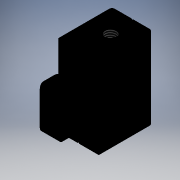
# Autodesk Inventor part: HCBRB8
Saved by Autodesk Inventor 2017.3 (Build 213256000, 256)
## iProperties
Part Number: HCBRB8
Material: Generic
Catalog Web Link: www.cadenas.de
Description: HCBR, HCBRB-Panel Support Brackets - Resin Type - for Center Mounting (One-Touch Mounting)
Vendor: MISUMI
Document SubType Name: Modeling
Designer: partserver
Manufacturer: MISUMI
Mass: 8.4889 g
Surface Area: 43.6631 cm^2
Volume: 8.4889 cm^3
Density: 1 g/cm^3
Appearance: PSOLRGB-0-0-0
Category: PARTsolutions
Company: MISUMI
Title: HCBRB8
Author: Cadenas PARTsolutions
Comments: Panel Support Brackets - Resin Type - for Center Mounting (One-Touch Mounting)
PSOL_IDENT_0: {$CADENAS_DATA\23d-libs\misumi\metric\39_accessories_for_al_extrusions\hcbr.prj},162 {VTYP=3D},{NB=H
PSOL_IDENT_1: CBRB8},{LINA=HCBRB8},{NN=HCBR, HCBRB},{DATE=08.06.2021 06:07:33},{GEOMDATE=12.08.2016 06:28:00},{VER
PSOL_IDENT_2: SION=},{LINEID=40},{WBVAR=COLOR},{WBNUMERIC=}  {NB=HCBRB8},{LINA=HCBRB8},{KT=DUMMY},{PN=HCBRB8},{COL
PSOL_IDENT_3: OR=B},{TS=HCBR},{MAT=Polyamide},{NO=8},{MASS=10.9},{A=30},{DIFF=5},{COL=0.00,0.00,0.00,0.00},{M=5},{
PSOL_IDENT_4: KDM=4.134}
NB: HCBRB8
NN: HCBR, HCBRB
NT: Panel Support Brackets - Resin Type - for Center Mounting (One-Touch Mounting)
NBSYN: $PN.
LINA: HCBRB8
CATALOG: Misumi
PN: HCBRB8
COLOR: Black
MAT: Polyamide
NO: 8
MASS: 10.9
A: 30
DIFF: 5
SUPPLIER: MISUMI
ARTICLENO: HCBRB8
BOMINFO: HCBRB8
CREATOR: CADENAS GmbH
Autodesk Inventor part; units mm, degrees
ref_plane "YZ Plane" through (0, 0, 0) normal (1, 0, 0) x (0, 1, 0)
ref_plane "XZ Plane" through (0, 0, 0) normal (0, 1, 0) x (-1, 0, 0)
ref_plane "XY Plane" through (0, 0, 0) normal (0, 0, 1) x (1, 0, 0)
sketch "Sketch_1" plane through (0, 0, 0) normal (0, 0, 1) x (1, 0, 0)
  line L0 (0, 28.85) -> (0, 9.95)
  line L1 (0, 9.95) -> (15, 9.95)
  line L2 (15, 9.95) -> (15, 28.85)
  arc A0 (15, 28.85) -> (14, 29.85) centre (14, 28.85) ccw
  line L3 (14, 29.85) -> (1, 29.85)
  arc A1 (1, 29.85) -> (0, 28.85) centre (1, 28.85) ccw
  constraints: 8 end point, 4 point on circle, 2 centre point
extrude "Extrusion1" add sketch "Sketch_1" against normal blind 30
sketch "Sketch_6" plane through (7.5, 0, 0) normal (1, 0, 0) x (0, 0, -1)
  line L0 (0, 21.4) -> (35, 21.4)
  line L1 (35, 21.4) -> (35, 18.15)
  line L2 (35, 18.15) -> (34.5, 18.65)
  line L3 (34.5, 18.65) -> (0.5, 18.65)
  line L4 (0.5, 18.65) -> (0, 18.15)
  line L5 (0, 18.15) -> (0, 21.4)
  line L6 (0, 21.4) -> (35, 21.4)
  constraints: 14 end point
revolve "Revolution1" cut sketch "Sketch_6" angle 360 about axis through (7.5, 21.4, 0) along (0, 0, 1)
sketch "Sketch_4" plane through (7.5, 0, 0) normal (1, 0, 0) x (0, 0, -1)
  line L0 (0, 22.5) -> (35, 22.5)
  line L1 (35, 22.5) -> (35, 19.25)
  line L2 (35, 19.25) -> (34.5, 19.75)
  line L3 (34.5, 19.75) -> (0.5, 19.75)
  line L4 (0.5, 19.75) -> (0, 19.25)
  line L5 (0, 19.25) -> (0, 22.5)
  line L6 (0, 22.5) -> (35, 22.5)
  constraints: 14 end point
revolve "Revolution2" cut sketch "Sketch_4" angle 360 about axis through (7.5, 22.5, 0) along (0, 0, 1)
sketch "Sketch_8" plane through (0, 21.95, 0) normal (0, 1, 0) x (1, 0, 0)
  line L0 (4.25, 0) -> (10.75, 0)
  line L1 (10.75, 0) -> (10.25, 0.5)
  line L2 (10.25, 0.5) -> (10.25, 34.5)
  line L3 (10.25, 34.5) -> (10.75, 35)
  line L4 (10.75, 35) -> (4.25, 35)
  line L5 (4.25, 35) -> (4.75, 34.5)
  line L6 (4.75, 34.5) -> (4.75, 0.5)
  line L7 (4.75, 0.5) -> (4.25, 0)
  constraints: 16 end point
extrude "Extrusion2" cut sketch "Sketch_8" along normal mid plane 1.1
sketch "Sketch_10" plane through (0, 0, -0.5) normal (0, 0, 1) x (1, 0, 0)
  arc A0 (4.75, 21.4) -> (10.25, 21.4) centre (7.5, 21.4) ccw
  line L0 (10.25, 21.4) -> (10.25, 22.5)
  arc A1 (10.25, 22.5) -> (4.75, 22.5) centre (7.5, 22.5) ccw
  line L1 (4.75, 22.5) -> (4.75, 21.4)
  constraints: 4 end point, 4 point on circle, 2 centre point
extrude "Extrusion3" add sketch "Sketch_10" against normal blind 29
sketch "Sketch_11" plane through (7.5, 0, 0) normal (1, 0, 0) x (0, 0, -1)
  line L0 (0.5, 21.95) -> (29.5, 21.95)
  line L1 (29.5, 21.95) -> (29.5, 19.45)
  line L2 (29.5, 19.45) -> (29.067, 19.883)
  line L3 (29.067, 19.883) -> (0.933, 19.883)
  line L4 (0.933, 19.883) -> (0.5, 19.45)
  line L5 (0.5, 19.45) -> (0.5, 21.95)
  line L6 (0.5, 21.95) -> (29.5, 21.95)
  constraints: 14 end point
revolve "Revolution3" cut sketch "Sketch_11" angle 360 about axis through (7.5, 21.95, -0.5) along (0, 0, 1)
thread "Thread1" size "M5x0.8" class "6H" standard "ISO Metric profile" full length
sketch "_____2" plane through (0, 9.95, 0) normal (0, 1, 0) x (1, 0, 0)
  line L0 (2.75, 17.75) -> (2.75, 14.75)
  arc A0 (2.75, 14.75) -> (7.25, 10.25) centre (7.25, 14.75) ccw
  line L1 (7.25, 10.25) -> (10.25, 10.25)
  arc A1 (10.25, 10.25) -> (12.25, 12.25) centre (10.25, 12.25) ccw
  line L2 (12.25, 12.25) -> (12.25, 15.25)
  arc A2 (12.25, 15.25) -> (7.75, 19.75) centre (7.75, 15.25) ccw
  line L3 (7.75, 19.75) -> (4.75, 19.75)
  arc A3 (4.75, 19.75) -> (2.75, 17.75) centre (4.75, 17.75) ccw
  constraints: 8 end point, 8 point on circle, 4 centre point
extrude "Extrusion4" add sketch "_____2" against normal blind 9.6
sketch "_____3" plane through (7.5, 0, 0) normal (1, 0, 0) x (0, 0, -1)
  line L0 (5.5, 4.65) -> (5.5, 2.35)
  arc A0 (5.5, 2.35) -> (7.5, 0.35) centre (7.5, 2.35) ccw
  line L1 (7.5, 0.35) -> (22.5, 0.35)
  arc A1 (22.5, 0.35) -> (24.5, 2.35) centre (22.5, 2.35) ccw
  line L2 (24.5, 2.35) -> (24.5, 4.65)
  line L3 (24.5, 4.65) -> (5.5, 4.65)
  constraints: 8 end point, 4 point on circle, 2 centre point
extrude "Extrusion5" add sketch "_____3" along normal mid plane 9.5
sketch "_____4" plane through (0, 0, -14.75) normal (0, 0, 1) x (1, 0, 0)
  line L0 (2.75, 4.25) -> (7.5, 4.65)
  line L1 (7.5, 4.65) -> (2.75, 4.65)
  line L2 (2.75, 4.65) -> (2.75, 4.25)
  constraints: 6 end point
extrude "Extrusion6" cut sketch "_____4" along normal blind 9.5
sketch "_____5" plane through (0, 0, -15.25) normal (0, 0, 1) x (1, 0, 0)
  line L0 (7.5, 4.65) -> (12.25, 4.25)
  line L1 (12.25, 4.25) -> (12.25, 4.65)
  line L2 (12.25, 4.65) -> (7.5, 4.65)
  constraints: 6 end point
extrude "Extrusion7" cut sketch "_____5" against normal blind 9.5
sketch "_____7" plane through (0, 0.35, 0) normal (0, 1, 0) x (1, 0, 0)
  line L0 (2.75, 17.75) -> (2.75, 14.75)
  arc A0 (2.75, 14.75) -> (7.25, 10.25) centre (7.25, 14.75) ccw
  line L1 (7.25, 10.25) -> (10.25, 10.25)
  arc A1 (10.25, 10.25) -> (12.25, 12.25) centre (10.25, 12.25) ccw
  line L2 (12.25, 12.25) -> (12.25, 15.25)
  arc A2 (12.25, 15.25) -> (7.75, 19.75) centre (7.75, 15.25) ccw
  line L3 (7.75, 19.75) -> (4.75, 19.75)
  arc A3 (4.75, 19.75) -> (2.75, 17.75) centre (4.75, 17.75) ccw
  constraints: 8 end point, 8 point on circle, 4 centre point
extrude "Extrusion8" add sketch "_____7" along normal blind 4.3
sketch "_____1" plane through (0, 0.35, 0) normal (0, 1, 0) x (1, 0, 0)
  line L0 (-10.5888, -9.9588) -> (25.3573, -9.9588)
  line L1 (25.3573, -9.9588) -> (25.3573, 39.1524)
  line L2 (25.3573, 39.1524) -> (-10.5888, 39.1524)
  line L3 (-10.5888, 39.1524) -> (-10.5888, -9.9588)
  arc A0 (2.75, 10.3) -> (7.55, 5.5) centre (7.55, 10.3) ccw
  line L4 (7.55, 5.5) -> (12.25, 5.5)
  line L5 (12.25, 5.5) -> (12.25, 19.7)
  arc A1 (12.25, 19.7) -> (7.45, 24.5) centre (7.45, 19.7) ccw
  line L6 (7.45, 24.5) -> (2.75, 24.5)
  line L7 (2.75, 24.5) -> (2.75, 10.3)
  constraints: 16 end point, 4 point on circle, 2 centre point
extrude "Extrusion9" cut sketch "_____1" along normal mid plane 19.2
sketch "Sketch_3" plane through (7.5, 0, 0) normal (1, 0, 0) x (0, 0, -1)
  line L0 (15, 0.35) -> (15, -1.45)
  line L1 (15, -1.45) -> (14.5, -1.45)
  line L2 (14.5, -1.45) -> (13, 0.35)
  line L3 (13, 0.35) -> (15, 0.35)
  line L4 (15, 0.35) -> (15, -1.45)
  constraints: 10 end point
revolve "Revolution4" add sketch "Sketch_3" angle 360 about axis through (7.5, 0.35, -15) along (0, 1, 0)
sketch "Sketch_7" plane through (15, 0, 0) normal (1, 0, 0) x (0, 0, -1)
  line L0 (2, 15.2) -> (2, 11.95)
  line L1 (2, 11.95) -> (14, 11.95)
  line L2 (14, 11.95) -> (14, 15.2)
  line L3 (14, 15.2) -> (2, 15.2)
  constraints: 8 end point
extrude "Extrusion10" cut sketch "Sketch_7" against normal blind 15
sketch "Sketch_5" plane through (15, 0, 0) normal (1, 0, 0) x (0, 0, -1)
  line L0 (16, 15.2) -> (16, 11.95)
  line L1 (16, 11.95) -> (28, 11.95)
  line L2 (28, 11.95) -> (28, 15.2)
  line L3 (28, 15.2) -> (16, 15.2)
  constraints: 8 end point
extrude "Extrusion11" cut sketch "Sketch_5" against normal blind 15
sketch "Sketch_9" plane through (0, 0, 0) normal (0, 1, 0) x (-1, 0, 0)
  line L0 (0, -15.3) -> (0, -14.7)
  line L1 (0, -14.7) -> (-0.3, -15)
  line L2 (-0.3, -15) -> (0, -15.3)
  constraints: 6 end point
extrude "Extrusion12" cut sketch "Sketch_9" along normal blind 40
sketch "Sketch_15" plane through (0, 0, 0) normal (0, 1, 0) x (-1, 0, 0)
  line L0 (-14.7, -15) -> (-15, -14.7)
  line L1 (-15, -14.7) -> (-15, -15.3)
  line L2 (-15, -15.3) -> (-14.7, -15)
  constraints: 6 end point
extrude "Extrusion13" cut sketch "Sketch_15" along normal blind 40
sketch "Sketch_16" plane through (0, 0, 0) normal (0, 1, 0) x (-1, 0, 0)
  line L0 (-7.2, 0) -> (-7.8, 0)
  line L1 (-7.8, 0) -> (-7.5, -0.3)
  line L2 (-7.5, -0.3) -> (-7.2, 0)
  constraints: 6 end point
extrude "Extrusion14" cut sketch "Sketch_16" along normal blind 40
sketch "Sketch_17" plane through (0, 0, 0) normal (0, 1, 0) x (-1, 0, 0)
  line L0 (-7.2, -30) -> (-7.5, -29.7)
  line L1 (-7.5, -29.7) -> (-7.8, -30)
  line L2 (-7.8, -30) -> (-7.2, -30)
  constraints: 6 end point
extrude "Extrusion15" cut sketch "Sketch_17" along normal blind 50
body "Solid1"
